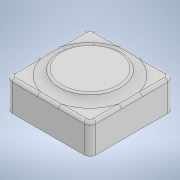
# Autodesk Inventor part: Small_Button
Saved by Autodesk Inventor 2021 (Build 250183000, 183)
## iProperties
Created: 2020-05-31
Part Number: Small_Button
Material: Generic
Document SubType Name: Modeling
Designer: ameli
Density: 1 g/cm^3
Appearance: Default
Author: ameli
Autodesk Inventor part; units mm, degrees
ref_plane "YZ Plane" through (0, 0, 0) normal (1, 0, 0) x (0, 1, 0)
ref_plane "XZ Plane" through (0, 0, 0) normal (0, 1, 0) x (-1, 0, 0)
ref_plane "XY Plane" through (0, 0, 0) normal (0, 0, 1) x (1, 0, 0)
sketch "Sketch5" plane through (0, 0, 0) normal (0, 1, 0) x (-1, 0, 0)
  line L0 (0, 0) -> (14, 0)
  line L1 (14, 0) -> (14, -14)
  line L2 (14, -14) -> (0, -14)
  line L3 (0, -14) -> (0, 0)
  dimension "d3" = 14
  dimension "d4" = 14
  constraints: 8 end point, 2 parallel, 1 horizontal, 1 perpendicular
  measures "d3" distance of L1.end L2.end
  measures "d4" distance of L0.end L1.end
extrude "Extrusion1" add sketch "Sketch5" along normal blind 5
sketch "Sketch6" plane through (0, 5, 0) normal (0, 1, 0) x (1, 0, 0)
  circle A0 centre (-7, 7) radius 5
  line L0 (0, 0) -> (0, 14) projected
  line L1 (0, 14) -> (-14, 14) projected
  dimension "d7" = 10
  dimension "d8" = 7
  dimension "d9" = 7
  constraints: 1 centre point
  measures "d7" diameter of A0
  measures "d8" distance from line of L0 A0.centre
  measures "d9" distance from line of L1 A0.centre
extrude "Extrusion2" add sketch "Sketch6" along normal blind 1
fillet "Fillet1" radius 2 1 edges at (-12, 5, -7)
fillet "Fillet2" radius 1 4 edges at (-14, 2.5, 0) (0, 2.5, 0) (-14, 2.5, -14) (0, 2.5, -14)
fillet "Fillet3" radius 0.5 9 edges at (-12, 6, -7) (-0.2929, 5, -13.7071) (-7, 5, -14) (-13.7071, 5, -13.7071) (-14, 5, -7) (-13.7071, 5, -0.2929) (-7, 5, 0) (-0.2929, 5, -0.2929) (0, 5, -7)
shell "Shell1" thickness 1.5 removed faces 1 at (-9, 0, -9.3333)
ref_plane "Work Plane2" through (-7, 0, -1) normal (1, 0, 0) x (0, 0, -1)
sketch "Sketch24" plane through (-7, 4.5, -7) normal (0, -1, 0) x (1, 0, 0)
  line L0 (-2.9999, 3.0001) -> (3.0001, 3.0001)
  line L1 (3.0001, 3.0001) -> (3.0001, -2.9999)
  line L2 (3.0001, -2.9999) -> (-2.9999, -2.9999)
  line L3 (-2.9999, -2.9999) -> (-2.9999, 3.0001)
  circle A0 centre (0, 0) radius 4.2826 projected
  point P0 (7, 7)
  dimension "d41" = 6
  dimension "d42" = 6
  dimension "d43" = 1.2825
  dimension "d44" = 1.2825
  constraints: 8 end point, 2 parallel, 1 horizontal, 1 perpendicular
  measures "d41" distance of L0.end L1.end
  measures "d42" distance of L0.start L0.end
  measures "d43" distance edge to line of A0 L1
  measures "d44" distance edge to line of A0 L0
extrude "Extrusion5" cut sketch "Sketch24" against normal blind 1 contours L0 L1 L2 L3
body "Solid1"
